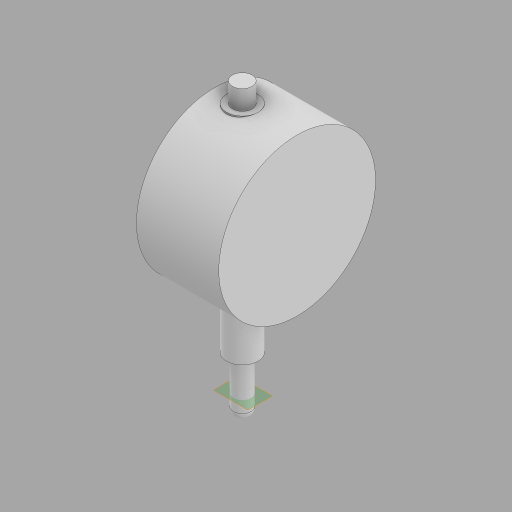
# Autodesk Inventor part: Messuhr-Dummy
Saved by Autodesk Inventor 2023 (Build 270158000, 158)
## iProperties
Created: 2024-12-10
Part Number: Messuhr-Dummy
Material: Generisch
Document SubType Name: Modeling
Designer: Nils Bade
Density: 1 g/cm^3
Appearance: Vorgabe
Author: Nils Bade
Autodesk Inventor part; units mm, degrees
ref_plane "YZ Plane" through (0, 0, 0) normal (1, 0, 0) x (0, 1, 0)
ref_plane "XZ Plane" through (0, 0, 0) normal (0, 1, 0) x (-1, 0, 0)
ref_plane "XY Plane" through (0, 0, 0) normal (0, 0, 1) x (1, 0, 0)
sketch "S-Pinout" plane through (0, 0, 0) normal (0, 1, 0) x (-1, 0, 0)
  circle A0 centre (0, 0) radius 4
  circle A1 centre (0, 0) radius 2.25
  dimension "d0" = 8
  dimension "d3" = 4.5
  constraints: 2 centre point, 2 coincident
  measures "d0" diameter of A0
  measures "d3" diameter of A1
extrude "Ex-passstift" add sketch "S-Pinout" along normal blind 40 and the other way blind 15 contours A0 | A1
extrude "Ex-Pin" add sketch "S-Pinout" against normal blind 14 from surface at -15 contours A1
fillet "Rundung-Pin" radius 2 1 edges at (2.25, -29, 0)
sketch "Skizze2" plane through (0, 0, 0) normal (1, 0, 0) x (0, 1, 0)
  circle A0 centre (20, 0) radius 20
  line L0 (-8, 0) -> (48, 0) construction
  line L1 (0, 28) -> (0, -28) projected
  point P0 (0, 0)
  dimension "d7" = 40
  constraints: 1 centre point, 1 midpoint, 1 tangent
  measures "d7" diameter of A0
extrude "Ex-Uhr" add sketch "Skizze2" along normal blind 14 and the other way blind 7
sketch "Skizze3" plane through (0, 40, 0) normal (0, 1, 0) x (1, 0, 0)
  circle A0 centre (0, 0) radius 0.25 projected
  circle A1 centre (0, 0) radius 2.5
  dimension "d14" = 5
  constraints: 1 centre point, 1 coincident
  measures "d14" diameter of A1
extrude "Ex-Taste" add sketch "Skizze3" along normal blind 5 contours A0 | A1
ref_plane "Messbereich" through (0, -24, 0) normal (0, -1, 0) x (1, 0, 0)
